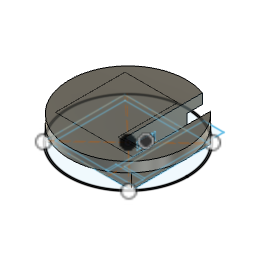
Drone_Station (Autodesk Fusion 360 design; units mm, degrees)
Autodesk Fusion 360 part; units mm, degrees
sketch "Esboço1" plane through (0, 0, 0) normal (0, 0, 1) x (1, 0, 0)
  circle A0 centre (0, 0) radius 120
  line L0 (85.6634, -84.0344) -> (-85.6634, 84.0344) construction
  line L1 (-85.6634, -84.0344) -> (85.6634, 84.0344) construction
  circle A1 centre (0, 0) radius 117.5
  line L2 (86.4532, -79.5744) -> (-86.4532, -79.5744)
  line L3 (-86.4532, -79.5744) -> (-86.4532, 79.5744)
  line L4 (-86.4532, 79.5744) -> (86.4532, 79.5744)
  line L5 (86.4532, 79.5744) -> (86.4532, -79.5744)
  line L6 (86.4532, -79.5744) -> (-86.4532, 79.5744) construction
  line L7 (-86.4532, -79.5744) -> (86.4532, 79.5744) construction
  line L8 (38.7429, 113.5737) -> (78.7429, 113.5737)
  line L9 (78.7429, 113.5737) -> (78.7429, -45.7782)
  line L10 (78.7429, -45.7782) -> (38.7429, -45.7782)
  line L11 (38.7429, -45.7782) -> (38.7429, 113.5737)
  line L12 (38.7429, 79.5744) -> (-86.4532, 79.5744) construction
  line L13 (-86.4532, 79.5744) -> (-86.4532, -79.5744) construction
  line L14 (-86.4532, -79.5744) -> (38.7429, -79.5744) construction
  line L15 (38.7429, -79.5744) -> (38.7429, 79.5744) construction
  line L16 (38.7429, 78.6764) -> (-86.6324, 78.6764) construction
  line L17 (-86.6324, 78.6764) -> (-86.6324, -79.3836) construction
  line L18 (-86.6324, -79.3836) -> (38.7429, -79.3836) construction
  line L19 (38.7429, -79.3836) -> (38.7429, 78.6764) construction
  line L20 (30.085, 69.8635) -> (-75.9118, 69.8635)
  line L21 (-75.9118, 69.8635) -> (-75.9118, -69.8718)
  line L22 (-75.9118, -69.8718) -> (30.085, -69.8718)
  line L23 (30.085, -69.8718) -> (30.085, 69.8635)
  line L24 (26.0377, -69.8718) -> (80, -69.8718)
  line L25 (80, -69.8718) -> (80, -50.192)
  line L26 (80, -50.192) -> (26.0377, -50.192)
  line L27 (26.0377, -50.192) -> (26.0377, -69.8718)
  dimension "d1" = 240
  dimension "d3" = 235
  dimension "d30" = 40
  constraint coincident A0.centre A1.centre
  constraint coincident L0 A0.centre
  constraint coincident L1 A0.centre
  constraint coincident A0 L0.end
  constraint concentric A0 A1
  constraint horizontal L2
  constraint perpendicular L2 L3
  constraint parallel L2 L4
  constraint parallel L3 L5
  constraint coincident L6 A0.centre
  constraint coincident L7 A0.centre
  constraint coincident A1 L3.end
  constraint horizontal L8
  constraint vertical L9
  constraint horizontal L10
  constraint vertical L11
  constraint coincident A0 L8.start
  constraint horizontal L12
  constraint vertical L13
  constraint horizontal L14
  constraint vertical L15
  constraint coincident L4 L12.start
  constraint coincident L11 L12.start
  constraint horizontal L16
  constraint vertical L17
  constraint horizontal L18
  constraint vertical L19
  constraint coincident L15 L16.start
  constraint horizontal L20
  constraint vertical L21
  constraint horizontal L22
  constraint vertical L23
  constraint coincident L7 L21.end
  constraint horizontal L24
  constraint vertical L25
  constraint horizontal L26
  constraint vertical L27
  constraint coincident L22 L24.start
  measures "d1" diameter of A0
  measures "d3" diameter of A1
  measures "d30" distance of L8.start L8.end
extrude "Extrusão1" add sketch "Esboço1" along normal blind 30 contours L2 L3 L4 L5 L9 L10 L11 | L4 L9 L10 L11 | L20 L21 L22 L23 L26 L27 | L23 L24 L25 L26 | L22 L23 L24 L26 L27
extrude "Extrusão2" add sketch "Esboço1" along normal blind 20 from surface at 30 contours A1 L4 L11 | A1 L4 L9 L11 | A1 L4 L9 | A1 L3 | L2 L3 L4 L5 L9 L10 L11 | L4 L9 L10 L11 | A1 L5 | A1 L2 | L20 L21 L22 L23 L26 L27 | L23 L24 L25 L26 | L22 L23 L24 L26 L27
extrude "Extrusão3" cut sketch "Esboço1" along normal up to surface (50 mm away) contours A1 L4 L9 L11 | L4 L9 L10 L11
sketch "Esboço2" plane through (38.7429, 0, 0) normal (1, 0, 0) x (0, 1, 0)
  line L0 (79.5744, 0) -> (79.5744, 30)
  line L1 (79.5744, 30) -> (110.929, 30)
  line L2 (110.929, 30) -> (110.929, 50)
  line L3 (110.929, 50) -> (-45.7782, 50)
  line L4 (-45.7782, 50) -> (-45.7782, 0)
  line L5 (-45.7782, 0) -> (79.5744, 0)
  line L6 (9.7973, 15.9746) -> (-15.2027, 15.9746)
  line L7 (-15.2027, 15.9746) -> (-15.2027, 29.9746)
  line L8 (-15.2027, 29.9746) -> (9.7973, 29.9746)
  line L9 (9.7973, 29.9746) -> (9.7973, 15.9746)
  line L10 (9.7973, 15.9746) -> (-15.2027, 29.9746) construction
  line L11 (-15.2027, 15.9746) -> (9.7973, 29.9746) construction
  line L12 (14.7973, 15.9746) -> (-20.2027, 15.9746)
  line L13 (-20.2027, 15.9746) -> (-20.2027, 29.9746)
  line L14 (-20.2027, 29.9746) -> (14.7973, 29.9746)
  line L15 (14.7973, 29.9746) -> (14.7973, 15.9746)
  line L16 (14.7973, 15.9746) -> (-20.2027, 29.9746) construction
  line L17 (-20.2027, 15.9746) -> (14.7973, 29.9746) construction
  point P0 (-2.7027, 22.9746)
  point P1 (-2.7027, 22.9746)
  point P2 (-2.7027, 22.9746)
  dimension "d20" = 25
  dimension "d22" = 14
  dimension "d23" = 35
  dimension "d24" = 14
  dimension "d25" = 14
  constraint horizontal L6
  constraint perpendicular L6 L7
  constraint parallel L6 L8
  constraint parallel L7 L9
  constraint coincident L10 P2
  constraint coincident L11 P2
  constraint coincident P2 P1
  constraint horizontal L12
  constraint perpendicular L12 L13
  constraint parallel L12 L14
  constraint parallel L13 L15
  constraint coincident L16 P2
  constraint coincident L17 P2
  measures "d20" distance of L6.start L6.end
  measures "d22" distance of L6.start L8.end
  measures "d23" distance of L13.end L14.end
  measures "d24" distance of L12.end L13.end
  measures "d25" distance of L6.end L7.end
extrude "Extrusão8" cut sketch "Esboço2" against normal blind 21 contours L6 L7 L8 L9 L12 L14
extrude "Extrusão9" cut sketch "Esboço1" along normal blind 49 contours L20 L21 L22 L23 L26 L27 | L23 L24 L25 L26 | L22 L23 L24 L26 L27
extrude "Extrusão10" cut sketch "Esboço2" against normal blind 2 contours L9 L12 L14 L15 | L7 L12 L13 L14
extrude "Extrusão4" [rolled back] along distance 20 taper angle 0
extrude "Extrusão5" [rolled back] along distance -20 taper angle 0
extrude "Extrusão6" [rolled back] along distance 1 taper angle 0
extrude "Extrusão7" [rolled back] along distance 39 taper angle 0
